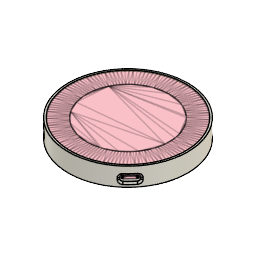
DisplayShell (Autodesk Fusion 360 design; units mm, degrees)
Autodesk Fusion 360 part; units mm, degrees
other "Base Mesh Feature1"
sketch "Sketch1" plane through (0, 0, 0) normal (0, 0, 1) x (1, 0, 0)
  circle A0 centre (0, 0) radius 36
  circle A1 centre (0, 0) radius 37.75
  circle A2 centre (0, 0) radius 39
  line L0 (10.5895, 34.4073) -> (-10.5895, 34.4073)
  line L1 (25.4504, -16.8148) -> (30.8083, -21.8155)
  line L2 (18.0508, -24.6231) -> (23.4041, -29.6194)
  line L3 (-17.4069, -24.414) -> (-23.2158, -29.7672)
  line L4 (-26.3415, -17.6187) -> (-30.8426, -21.7668)
  dimension "d1" = 72
  dimension "d2" = 75.5
  dimension "d3" = 78
  constraint coincident A0.centre A1.centre
  constraint concentric A0 A1
  constraint concentric A0 A2
  constraint coincident A0 L0.start
  constraint coincident A0 L0.end
  constraint horizontal L0
  constraint coincident A1 L1.end
  constraint coincident A1 L2.end
  constraint parallel L1 L2
  constraint coincident A1 L3.end
  constraint coincident A1 L4.end
  constraint parallel L3 L4
  measures "d1" diameter of A0
  measures "d2" diameter of A1
  measures "d3" diameter of A2
other "Modify1"
extrude "Extrude1" add sketch "Sketch1" against normal blind 9 contours A0 A1 L1 L4 | A0 A1 L2 L3 makes body 1 at (-32.8088, -18.6721, -6) makes body 2 at (-16.9338, -33.7388, -3)
extrude "Extrude2" add sketch "Sketch1" against normal blind 10 separate body makes body 3
move_body "Move1" bodies 3 to x (1, 0, 0) y (0, 1, 0) z (0, 0, 1) at (0, 0, 1)
extrude "Extrude3" add sketch "Sketch1" against normal blind 9 contours A0 L0 picked at (1.7848, 34.8047) bodies 1
ref_plane "WorkPlane1" through (0, 0, 12.125) normal (-0.71934, 0.694658, 0) x (0, 0, 1)
sketch "Sketch5" plane through (0, 0, 0) normal (-0.71934, 0.694658, 0) x (0, 0, 1)
  line L0 (-5.804, 5.1483) -> (-6.9533, 5.1483)
  line L1 (-8.4533, 3.6483) -> (-8.4533, -3.0079)
  line L2 (-6.9533, -4.5079) -> (-5.804, -4.5079)
  line L3 (-4.304, -3.0079) -> (-4.304, 3.6483)
  arc A0 (-6.9533, 5.1483) -> (-8.4533, 3.6483) centre (-6.9533, 3.6483) ccw
  arc A1 (-4.304, 3.6483) -> (-5.804, 5.1483) centre (-5.804, 3.6483) ccw
  arc A2 (-8.4533, -3.0079) -> (-6.9533, -4.5079) centre (-6.9533, -3.0079) ccw
  arc A3 (-5.804, -4.5079) -> (-4.304, -3.0079) centre (-5.804, -3.0079) ccw
  dimension "d11" = 1.5
  dimension "d12" = 1.5
  dimension "d13" = 1.5
  dimension "d14" = 1.5
  constraint horizontal L0
  constraint vertical L1
  constraint horizontal L2
  constraint vertical L3
  constraint tangent L0 A0
  constraint tangent L1 A0
  constraint tangent L0 A1
  constraint tangent L3 A1
  constraint tangent L2 A2
  constraint tangent L1 A2
  constraint tangent L2 A3
  constraint tangent L3 A3
  measures "d11" radius of A0
  measures "d12" radius of A1
  measures "d13" radius of A2
  measures "d14" radius of A3
extrude "Extrude4" cut sketch "Sketch5" against normal blind 100 bodies 3
ref_plane "WorkPlane2" through (0, 0, 12.125) normal (0.71934, 0.694658, 0) x (0, 0, 1)
sketch "Sketch7" plane through (0, 0, 0) normal (0.71934, 0.694658, 0) x (0, 0, 1)
  arc A0 (-4.354, 2.8138) -> (-5.854, 4.3138) centre (-5.854, 2.8138) ccw
  line L0 (-5.854, 4.3138) -> (-7.0088, 4.3138)
  arc A1 (-7.0088, 4.3138) -> (-8.5088, 2.8138) centre (-7.0088, 2.8138) ccw
  line L1 (-8.5088, 2.8138) -> (-8.5088, -3.4687)
  arc A2 (-8.5088, -3.4687) -> (-7.0088, -4.9687) centre (-7.0088, -3.4687) ccw
  line L2 (-7.0088, -4.9687) -> (-5.854, -4.9687)
  arc A3 (-5.854, -4.9687) -> (-4.354, -3.4687) centre (-5.854, -3.4687) ccw
  line L3 (-4.354, -3.4687) -> (-4.354, 2.8138)
  dimension "d18" = 1.5
  dimension "d19" = 1.5
  dimension "d20" = 1.5
  dimension "d21" = 1.5
  constraint horizontal L0
  constraint vertical L1
  constraint horizontal L2
  constraint vertical L3
  constraint tangent L0 A1
  constraint tangent A1 L1
  constraint tangent A0 L0
  constraint tangent A0 L3
  constraint tangent A2 L2
  constraint tangent L1 A2
  constraint tangent L2 A3
  constraint tangent A3 L3
  measures "d18" radius of A1
  measures "d19" radius of A0
  measures "d20" radius of A2
  measures "d21" radius of A3
extrude "Extrude6" cut sketch "Sketch7" against normal blind 100 bodies 3
ref_plane "WorkPlane3" through (0, 0, 12.125) normal (-0.642788, 0.766044, 0) x (0, 0, 1)
sketch "Sketch8" plane through (0, 0, 0) normal (-0.642788, 0.766044, 0) x (0, 0, 1)
  line L0 (-6.6037, 5.4228) -> (-4.68, 5.4228)
  line L1 (-4.18, 4.9228) -> (-4.18, -9.5289)
  line L2 (-4.68, -10.0289) -> (-6.6037, -10.0289)
  line L3 (-7.1037, -9.5289) -> (-7.1037, 4.9228)
  arc A0 (-6.6037, 5.4228) -> (-7.1037, 4.9228) centre (-6.6037, 4.9228) ccw
  arc A1 (-4.18, 4.9228) -> (-4.68, 5.4228) centre (-4.68, 4.9228) ccw
  arc A2 (-4.68, -10.0289) -> (-4.18, -9.5289) centre (-4.68, -9.5289) ccw
  arc A3 (-7.1037, -9.5289) -> (-6.6037, -10.0289) centre (-6.6037, -9.5289) ccw
  dimension "d27" = 0.5
  constraint horizontal L0
  constraint vertical L1
  constraint horizontal L2
  constraint vertical L3
  constraint tangent L3 A0
  constraint tangent L0 A0
  constraint tangent L0 A1
  constraint tangent L1 A1
  constraint equal A0 A1
  constraint tangent L1 A2
  constraint tangent L2 A2
  constraint equal A0 A2
  constraint tangent L2 A3
  constraint tangent L3 A3
  constraint equal A0 A3
  measures "d27" radius of A0
extrude "Extrude7" cut sketch "Sketch8" along normal blind 100 bodies 1 3
extrude "Extrude8" add sketch "Sketch1" along normal blind 2 separate body contours A0 L0 | A0 A1 L1 L4 | A0 L0 | A0 A1 L1 L2 | A0 A1 L2 L3 | A0 A1 L3 L4 | A2 makes body 4
move_body "Move2" bodies 4 to x (1, 0, 0) y (0, 1, 0) z (0, 0, 1) at (0, 0, -11)
combine "Combine2" operation add target body 3 tool bodies 1 2 4
fillet "Fillet1" radius 0.75 8 edges at (-31.9083, 22.4246, -5.6419) (-31.8195, 22.5504, -6.9597) (-26.8189, 28.3152, -7.1037) (-20.7969, 32.9923, -6.9579) (-20.6711, 33.0712, -5.6419) (-20.7969, 32.9923, -4.3258) (-26.8189, 28.3152, -4.18) (-31.8195, 22.5504, -4.3241) on bodies 3
fillet "Fillet2" radius 1 5 edges at (-31.2772, -23.2967, -6.4314) (-31.0101, -23.651, -4.7922) (-28.2814, -26.8544, -4.354) (-25.2246, -29.7443, -4.7926) (-24.8855, -30.0286, -6.4314) on bodies 3
fillet "Fillet3" radius 1 5 edges at (24.7347, -30.1528, -6.3786) (25.0755, -29.87, -4.7425) (28.2765, -26.8596, -4.304) (31.1194, -23.5071, -4.7421) (31.385, -23.1512, -6.3786) on bodies 3
hole "Hole1" at (-18.0769, -27.134, -11) direction (0, 0, 1) diameter 3 depth 10 tip angle 180 countersink diameter 5 countersink angle 90 bodies 3
hole "Hole2" at (-29.5447, 13.5918, -11) direction (0, 0, 1) diameter 3 depth 10 tip angle 180 countersink diameter 5 countersink angle 90 bodies 3
hole "Hole3" at (29.5117, 13.6063, -11) direction (0, 0, 1) diameter 3 depth 10 tip angle 180 countersink diameter 5 countersink angle 90 bodies 3
hole "Hole4" at (17.9628, -27.0689, -11) direction (0, 0, 1) diameter 3 depth 10 tip angle 180 countersink diameter 5 countersink angle 90 bodies 3
sketch "Sketch10" plane through (0, 0, -11) normal (0, 0, -1) x (1, 0, 0)
  circle A0 centre (17.9628, 27.0689) radius 2.5
  circle A1 centre (29.5117, -13.6063) radius 2.5
  circle A2 centre (-29.5447, -13.5918) radius 2.5
  circle A3 centre (-18.0769, 27.134) radius 2.5
  circle A4 centre (0, 0) radius 39
  circle A5 centre (0, 0) radius 15
  circle A6 centre (0, 0) radius 25
  line L0 (-5.003, 24.4943) -> (-4.7393, 24.4943)
  line L1 (-4.7393, 14.2316) -> (-5.003, 14.2316)
  line L2 (5.003, 24.4943) -> (5.0568, 24.4943)
  line L3 (5.0568, 14.1219) -> (5.003, 14.1219)
  line L4 (-4.841, -14.1973) -> (-5.0837, -14.1973)
  line L5 (-5.0837, -24.4777) -> (-4.841, -24.4777)
  line L6 (5.003, -14.1411) -> (5.0837, -14.1411)
  line L7 (5.0837, -24.4777) -> (5.003, -24.4777)
  line L8 (24.5275, -4.8273) -> (24.5275, -4.8376)
  line L9 (14.202, -4.8376) -> (14.202, -4.8273)
  line L10 (24.5275, 4.8273) -> (24.5275, 4.8376)
  line L11 (14.202, 4.8376) -> (14.202, 4.8273)
  line L12 (0, 0) -> (21.6506, 12.5)
  line L13 (0, 0) -> (25, 0) construction
  line L14 (0, 0) -> (21.6506, -12.5)
  line L15 (0, 0) -> (25, 0) construction
  line L16 (0, 0) -> (-21.6506, 12.5)
  line L17 (0, 0) -> (-21.6506, -12.5)
  dimension "d70" = 30
  dimension "d71" = 50
  dimension "d72" = 30
  dimension "d73" = 30
  constraint concentric A4 A5
  constraint concentric A5 A6
  constraint horizontal L0
  constraint horizontal L1
  constraint coincident A5 L1.start
  constraint coincident A6 L0.start
  constraint horizontal L2
  constraint horizontal L3
  constraint coincident A5 L3.start
  constraint coincident A6 L2.start
  constraint horizontal L4
  constraint horizontal L5
  constraint coincident A6 L5.start
  constraint coincident A5 L4.start
  constraint horizontal L6
  constraint horizontal L7
  constraint coincident A6 L7.start
  constraint coincident A5 L6.start
  constraint vertical L8
  constraint vertical L9
  constraint coincident A6 L8.end
  constraint coincident A5 L9.end
  constraint vertical L10
  constraint vertical L11
  constraint coincident A6 L10.end
  constraint coincident A5 L11.end
  constraint horizontal L13
  constraint coincident A4.centre A5.centre
  constraint horizontal L15
  constraint coincident A6 L14.end
  constraint coincident A6 L16.end
  constraint parallel L14 L16
  constraint coincident A6 L17.end
  measures "d70" diameter of A5
  measures "d71" diameter of A6
  measures "d72" angle of L12 L13
  measures "d73" angle of L14 L15
extrude "Extrude9" cut sketch "Sketch10" against normal blind 2 contours A5 A6 L12 L16 | A5 A6 L14 L17 bodies 3
